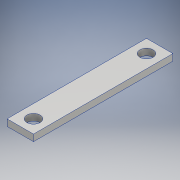
# Autodesk Inventor part: rocker_bogie_plate
Saved by Autodesk Inventor 2018.1 (Build 221171000, 171)
## iProperties
Created: 2017-10-26
Part Number: rocker_bogie_plate
Material: アルミニウム 6061
Document SubType Name: Modeling
Designer: Kakeru Yamashita
Density: 2.7 g/cm^3
Appearance: アルミニウム - フラット
Author: Kakeru Yamashita
Autodesk Inventor part; units mm, degrees
ref_plane "YZ Plane" through (0, 0, 0) normal (1, 0, 0) x (0, 1, 0)
ref_plane "XZ Plane" through (0, 0, 0) normal (0, 1, 0) x (-1, 0, 0)
ref_plane "XY Plane" through (0, 0, 0) normal (0, 0, 1) x (1, 0, 0)
sketch "スケッチ1" plane through (0, 0, 0) normal (0, 0, 1) x (1, 0, 0)
  line L0 (0, 0) -> (20, 0)
  line L1 (20, 0) -> (20, 105.6)
  line L2 (20, 105.6) -> (0, 105.6)
  line L3 (0, 105.6) -> (0, 0)
  circle A0 centre (10, 95.6) radius 5
  circle A1 centre (10, 10) radius 5
  dimension "d0" = 20
  dimension "d1" = 105.6
  dimension "d2" = 10
  dimension "d3" = 10
  dimension "d4" = 10
  dimension "d5" = 10
  dimension "d6" = 10
  dimension "d7" = 10
  constraints: 8 end point, 2 centre point, 2 parallel, 1 horizontal, 1 perpendicular
  measures "d0" distance of L1.end L2.end
  measures "d1" distance of L0.end L1.end
  measures "d2" diameter of A0
  measures "d3" diameter of A1
  measures "d4" distance from line of L2 A0.centre
  measures "d5" distance from line of L3 A0.centre
  measures "d6" distance from line of L0 A1.centre
  measures "d7" distance from line of L3 A1.centre
extrude "押し出し1" add sketch "スケッチ1" along normal blind 5
